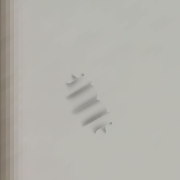
# Autodesk Inventor part: wrenchC
Saved by Autodesk Inventor 2017 (Build 210142000, 142)
## iProperties
Created: 2017-02-16
Part Number: wrenchC
Material: Generic
Document SubType Name: Modeling
Designer: kingb
Density: 1 g/cm^3
Appearance: Glossy - Black
Author: kingb
Autodesk Inventor part; units mm, degrees
ref_plane "YZ Plane" through (0, 0, 0) normal (1, 0, 0) x (0, 1, 0)
ref_plane "Work Plane1" through (0, 0, 0) normal (0, 0, 1) x (1, 0, 0)
sketch "Sketch1" plane through (0, 0, 0) normal (0, 0, 1) x (1, 0, 0)
  circle A0 centre (20.32, 4.1275) radius 11.176 projected
  circle A1 centre (20.32, 4.1275) radius 8.255
  arc A2 (18.415, 12.1597) -> (22.225, 12.1597) centre (20.32, 13.3688) ccw
  line L0 (22.225, 12.1597) -> (18.415, 12.1597)
  line L1 (9.144, 4.1275) -> (31.496, 4.1275) construction
  arc A3 (14.6541, 10.1311) -> (17.9537, 12.0361) centre (15.6993, 12.1307) ccw
  line L2 (17.9537, 12.0361) -> (14.6541, 10.1311)
  circle A4 centre (20.32, 4.1275) radius 8.255
  arc A5 (12.4114, 6.4938) -> (14.3164, 9.7934) centre (12.3168, 8.7482) ccw
  line L3 (14.3164, 9.7934) -> (12.4114, 6.4938)
  circle A6 centre (20.32, 4.1275) radius 8.255
  arc A7 (12.2878, 2.2225) -> (12.2878, 6.0325) centre (11.0787, 4.1275) ccw
  line L4 (12.2878, 6.0325) -> (12.2878, 2.2225)
  circle A8 centre (20.32, 4.1275) radius 8.255
  arc A9 (14.3164, -1.5384) -> (12.4114, 1.7612) centre (12.3168, -0.4932) ccw
  line L5 (12.4114, 1.7612) -> (14.3164, -1.5384)
  circle A10 centre (20.32, 4.1275) radius 8.255
  arc A11 (17.9537, -3.7811) -> (14.6541, -1.8761) centre (15.6993, -3.8757) ccw
  line L6 (14.6541, -1.8761) -> (17.9537, -3.7811)
  circle A12 centre (20.32, 4.1275) radius 8.255
  arc A13 (22.225, -3.9047) -> (18.415, -3.9047) centre (20.32, -5.1138) ccw
  line L7 (18.415, -3.9047) -> (22.225, -3.9047)
  circle A14 centre (20.32, 4.1275) radius 8.255
  arc A15 (25.9859, -1.8761) -> (22.6863, -3.7811) centre (24.9407, -3.8757) ccw
  line L8 (22.6863, -3.7811) -> (25.9859, -1.8761)
  circle A16 centre (20.32, 4.1275) radius 8.255
  arc A17 (28.2286, 1.7612) -> (26.3236, -1.5384) centre (28.3232, -0.4932) ccw
  line L9 (26.3236, -1.5384) -> (28.2286, 1.7612)
  circle A18 centre (20.32, 4.1275) radius 8.255
  arc A19 (28.3522, 6.0325) -> (28.3522, 2.2225) centre (29.5613, 4.1275) ccw
  line L10 (28.3522, 2.2225) -> (28.3522, 6.0325)
  circle A20 centre (20.32, 4.1275) radius 8.255
  arc A21 (26.3236, 9.7934) -> (28.2286, 6.4938) centre (28.3232, 8.7482) ccw
  line L11 (28.2286, 6.4938) -> (26.3236, 9.7934)
  circle A22 centre (20.32, 4.1275) radius 8.255
  arc A23 (22.6863, 12.0361) -> (25.9859, 10.1311) centre (24.9407, 12.1307) ccw
  line L12 (25.9859, 10.1311) -> (22.6863, 12.0361)
  circle A24 centre (20.32, 4.1275) radius 8.255
  point P0 (0, 0)
  dimension "d0" = 2.921
  dimension "d1" = 3.81
  dimension "d2" = 1.27
  dimension "d3" = 0
  dimension "d6" = 360
  constraints: 50 point on circle, 26 end point, 24 centre point, 2 coincident, 1 horizontal, 1 line through centre, 1 midpoint, 83 other
  measures "d0" radial gap between concentric circles of A0 A1
  measures "d1" distance of L0.start L0.end
  measures "d3" angle of L1 L0
ref_plane "Work Plane2" through (0, -8.3185, -8.636) normal (0, 0, -1) x (0, 1, 0)
extrude "Extrusion1" add sketch "Sketch1" against normal up to surface (8.636 mm away) contours A0 | A1 L10 | L10 A19 | L11 A1 | A21 L11 | L9 A17 | A1 L9 | L12 A1 | A23 L12 | L8 A15 | A1 L8 | L0 A1 | A2 L0 | L7 A13 | A1 L7 | L2 A1 | A3 L2 | L6 A11 | A1 L6 | L3 A1 | A5 L3 | L5 A9 | A1 L5 | L4 A1 | A7 L4
body "Solid1"
